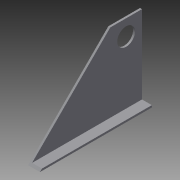
# Autodesk Inventor part: Z-Plate-R
Saved by Autodesk Inventor 2013 (Build 170138000, 138)
## iProperties
Created: 2014-01-24
Part Number: Z-Plate-R
Material: Generic
Document SubType Name: Modeling
Designer: Jarod
Density: 1 g/cm^3
Author: Jarod
Autodesk Inventor part; units mm, degrees
ref_plane "YZ Plane" through (0, 0, 0) normal (1, 0, 0) x (0, 1, 0)
ref_plane "XZ Plane" through (0, 0, 0) normal (0, 1, 0) x (-1, 0, 0)
ref_plane "XY Plane" through (0, 0, 0) normal (0, 0, 1) x (1, 0, 0)
sketch "Sketch1" plane through (0, 0, 0) normal (1, 0, 0) x (0, 1, 0)
  line L0 (0, 0) -> (103.2002, 0)
  line L1 (0, 0) -> (103.2002, 0) construction
  circle A0 centre (103.2002, 0) radius 14.2875
  line L2 (103.2002, 0) -> (128.6002, 0)
  line L3 (103.2002, 0) -> (128.6002, 0) construction
  line L4 (128.6002, 0) -> (128.6002, -25.4)
  line L5 (128.6002, -25.4) -> (0, -25.4)
  line L6 (0, -25.4) -> (0, 0)
  line L7 (128.6002, 0) -> (128.6002, 25.4)
  line L8 (128.6002, 0) -> (154.0002, 0) construction
  line L9 (128.6002, 25.4) -> (0, 154.0002)
  line L10 (0, 154.0002) -> (0, 0)
  dimension "d0" = 103.2002
  dimension "d1" = 0
  dimension "d2" = 28.575
  dimension "d3" = 25.4
  dimension "d4" = 0
  dimension "d5" = 25.4
  dimension "d6" = 90
  dimension "d7" = 25.4
  dimension "d8" = 90
  dimension "d9" = 135
  constraints: 22 end point, 4 horizontal, 3 equal length, 3 parallel, 1 centre point, 1 coincident, 1 collinear, 1 perpendicular
  measures "d0" distance of L0.start L0.end
  measures "d1" distance between parallel lines of L0 L1
  measures "d2" diameter of A0
  measures "d3" distance of L2.start L2.end
  measures "d4" distance between parallel lines of L2 L3
  measures "d5" distance of L3.end L4.end
  measures "d6" angle of L4 L5
  measures "d7" distance of L3.end L7.end
  measures "d8" angle of L8 L7
  measures "d9" angle of L9 L7
extrude "Extrusion1" add sketch "Sketch1" along normal blind 3.175 contours L10 L9 L7 L2 A0 L0 | L0 A0 L2 L4 L5 L6
sketch "Sketch2" plane through (3.175, 0, 0) normal (1, 0, 0) x (0, 0, -1)
  line L0 (-154.0002, 0) -> (25.4, 0) projected
  line L1 (25.4, 0) -> (25.4, 128.6002) projected
  line L2 (-25.4, 128.6002) -> (-154.0002, 0) projected
  line L3 (25.4, 0) -> (25.4, 3.175)
  line L4 (25.4, 0) -> (28.575, 0) construction
  line L5 (25.4, 3.175) -> (-150.8252, 3.175)
  point P0 (0, 0)
  dimension "d12" = 3.175
  dimension "d13" = 90
  constraints: 6 end point, 2 perpendicular, 1 collinear, 1 horizontal, 1 point on line
  measures "d12" distance of L0.end L3.end
  measures "d13" angle of L4 L3
extrude "Extrusion2" add sketch "Sketch2" along normal blind 15.875
body "Solid1"
